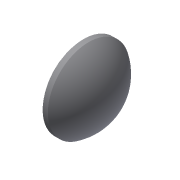
# Autodesk Inventor part: 00_lens_10mm
Saved by Autodesk Inventor 2019.4 (Build 234330000, 330)
## iProperties
Created: 2021-01-25
Part Number: 00_lens_10mm
Material: Generic
Document SubType Name: Modeling
Designer: diederichbenedict
Density: 1 g/cm^3
Appearance: Default
Author: diederichbenedict
Autodesk Inventor part; units mm, degrees
ref_plane "YZ Plane" through (0, 0, 0) normal (1, 0, 0) x (0, 1, 0)
ref_plane "XZ Plane" through (0, 0, 0) normal (0, 1, 0) x (-1, 0, 0)
ref_plane "XY Plane" through (0, 0, 0) normal (0, 0, 1) x (1, 0, 0)
sketch "Sketch1" plane through (0, 0, 0) normal (0, 1, 0) x (-1, 0, 0)
  line L0 (0, 0) -> (-4.8615, 0)
  arc A0 (0, 0) -> (-2.8, 7.86) centre (-12.4321, 0) ccw
  arc A1 (-3.8, 7.86) -> (-8.1, 0) centre (1.2337, 0) ccw
  line L1 (-2.8, 7.86) -> (-3.8, 7.86)
  line L2 (0, 0) -> (-8.1, 0)
  dimension "d0" = 8.1
  dimension "d1" = 2.8
  dimension "d2" = 7.86
  dimension "d3" = 1
  constraints: 6 end point, 4 point on circle, 2 centre point, 2 horizontal, 2 line through centre, 1 parallel, 1 point on line
  measures "d0" distance of L2.end L0.start
  measures "d1" horizontal distance of L1.start L0.start
  measures "d2" distance between parallel lines of L0 L1
  measures "d3" distance of L1.end L1.start
revolve "Revolution1" add sketch "Sketch1" angle 360 about axis through (0, 0, 0) along (1, 0, 0)
body "Solid1"
